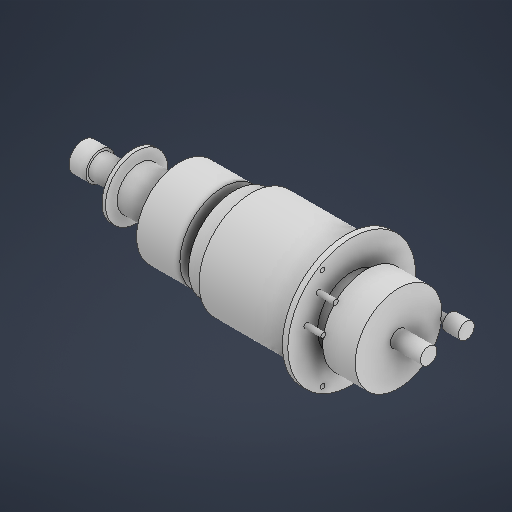
# Autodesk Inventor part: STI NGC Cryocooler
Saved by Autodesk Inventor 2026 (Build 300175050, 175E)
## iProperties
Created: 2024-04-30
Part Number: STI NGC Cryocooler
Material: Generic
Document SubType Name: Modeling
Designer: incep
Density: 1 g/cm^3
Appearance: Default
Author: incep
Autodesk Inventor part; units mm, degrees
ref_plane "YZ Plane" through (0, 0, 0) normal (1, 0, 0) x (0, 1, 0)
ref_plane "XZ Plane" through (0, 0, 0) normal (0, 1, 0) x (-1, 0, 0)
ref_plane "XY Plane" through (0, 0, 0) normal (0, 0, 1) x (1, 0, 0)
sketch "Sketch1" plane through (0, 0, 0) normal (0, 1, 0) x (-1, 0, 0)
  line L0 (0, 0) -> (-303.89, 0)
  line L1 (0, 0) -> (0, -10.5)
  line L2 (0, -10.5) -> (-94.6, -10.5)
  line L3 (-94.6, -10.5) -> (-94.6, -17.1)
  line L4 (-94.6, -17.1) -> (-46.4, -17.1)
  line L5 (-46.4, -17.1) -> (-46.4, -20.31)
  line L6 (-46.4, -20.31) -> (-43.9, -20.31)
  line L7 (-43.9, -20.31) -> (-43.9, -27.45)
  line L8 (-43.9, -27.45) -> (-47, -27.45)
  line L9 (-47, -27.45) -> (-48.9, -19.05)
  line L10 (-48.9, -19.05) -> (-84.8, -19.05)
  line L11 (-84.8, -19.05) -> (-84.8, -37.85)
  line L12 (-84.8, -37.85) -> (-122.9, -37.85)
  line L13 (-122.9, -37.85) -> (-122.9, -25.55)
  line L14 (-122.9, -25.55) -> (-132.9, -40.25)
  line L15 (-132.9, -40.25) -> (-132.9, -40.25)
  line L16 (-132.9, -40.25) -> (-147.9, -40.25)
  line L17 (-147.9, -40.25) -> (-147.9, -46)
  line L18 (-147.9, -46) -> (-150, -46)
  line L19 (-150, -46) -> (-150, -46)
  line L20 (-150, -46) -> (-231.4, -46)
  line L21 (-231.4, -46) -> (-231.4, -56.15)
  line L22 (-231.4, -56.15) -> (-236.2, -56.15)
  line L23 (-236.2, -56.15) -> (-236.2, 0)
  line L24 (-248.9, 0) -> (-248.9, -38.15)
  line L25 (-248.9, -38.15) -> (-277.4, -38.15)
  line L26 (-277.4, -38.15) -> (-277.4, -7.165)
  line L27 (-277.4, -7.165) -> (-303.89, -7.165)
  line L28 (-303.89, -7.165) -> (-303.89, 0)
  line L29 (0, -10.5) -> (0, -12.55)
  line L30 (0, -12.55) -> (-15, -12.55)
  line L31 (-15, -12.55) -> (-15, -10.5)
  line L32 (-236.2, 0) -> (-248.9, 0)
  line L33 (-248.9, 0) -> (-248.9, -30)
  line L34 (-248.9, -30) -> (-236.2, -30)
  line L35 (-236.2, -30) -> (-236.2, 0)
  dimension "d0" = 303.89
  dimension "d1" = 10.5
  dimension "d2" = 94.6
  dimension "d3" = 6.6
  dimension "d4" = 48.2
  dimension "d5" = 3.21
  dimension "d6" = 2.5
  dimension "d7" = 27.45
  dimension "d8" = 3.1
  dimension "d9" = 5
  dimension "d10" = 19.05
  dimension "d11" = 37.8
  dimension "d12" = 37.85
  dimension "d13" = 38.1
  dimension "d14" = 12.3
  dimension "d16" = 10
  dimension "d17" = 40.25
  dimension "d18" = 40.25
  dimension "d19" = 15
  dimension "d20" = 46
  dimension "d21" = 2.1
  dimension "d22" = 46
  dimension "d23" = 98.5
  dimension "d24" = 56.15
  dimension "d25" = 103.3
  dimension "d26" = 12.7
  dimension "d27" = 144.5
  dimension "d28" = 38.15
  dimension "d29" = 90
  dimension "d30" = 7.165
  dimension "d31" = 26.49
  dimension "d54" = 15
  dimension "d55" = 12.55
  dimension "d56" = 30
  constraints: 72 end point, 14 perpendicular, 9 vertical, 5 horizontal, 4 parallel, 4 point on line, 1 collinear
  measures "d0" distance of L0.start L0.end
  measures "d1" distance of L0.start L1.end
  measures "d2" distance of L1.end L2.end
  measures "d3" distance of L2.end L3.end
  measures "d4" distance of L3.end L4.end
  measures "d5" distance of L4.end L5.end
  measures "d6" distance of L5.end L6.end
  measures "d7" vertical distance of L0.start L7.end
  measures "d8" distance of L7.end L8.end
  measures "d9" distance from line of L9.end L7
  measures "d10" distance from line of L10 L0.start
  measures "d11" distance from line of L11 L8.end
  measures "d12" distance from line of L0.start L12
  measures "d13" distance of L11.end L12.end
  measures "d14" distance of L12.end L13.end
  measures "d16" distance between parallel lines of L15 L13
  measures "d17" distance from line of L14.end L0
  measures "d18" distance between parallel lines of L0 L16
  measures "d19" distance of L15.end L16.end
  measures "d20" distance between parallel lines of L0 L18
  measures "d21" distance of L17.end L18.end
  measures "d22" distance between parallel lines of L0 L20
  measures "d23" distance from line of L20.end L15
  measures "d24" distance between parallel lines of L0 L22
  measures "d25" distance between parallel lines of L23 L15
  measures "d26" distance between parallel lines of L24 L23
  measures "d27" distance from line of L25.end L15
  measures "d28" distance between parallel lines of L0 L25
  measures "d29" angle of L27 L26
  measures "d30" distance of L27.end L0.end
  measures "d31" distance of L26.end L27.end
  measures "d54" distance of L29.end L30.end
  measures "d55" distance between parallel lines of L0 L30
  measures "d56" distance between parallel lines of L34 L0
revolve "Revolution1" add sketch "Sketch1" angle 360 about axis through (0, 0, 0) along (1, 0, 0)
sketch "Sketch6" plane through (236.2, 0, 0) normal (1, 0, 0) x (0, 0, -1)
  line L0 (-25.5477, -44.25) -> (-25.5477, 44.25)
  line L1 (-25.5477, 44.25) -> (51.0955, 0)
  line L2 (51.0955, 0) -> (-25.5477, -44.25)
  circle A0 centre (51.0955, 0) radius 2
  circle A1 centre (-25.5477, -44.25) radius 2
  circle A2 centre (-25.5477, 44.25) radius 2
  point P0 (0, 0)
  point P1 (0, 0)
  dimension "d57" = 4
  dimension "d58" = 88.5
  constraints: 6 end point, 4 coincident, 3 centre point, 2 equal radius, 1 vertical, 7 other
  measures "d57" diameter of A0
  measures "d58" distance of L1.end L0.start
extrude "Extrusion3" cut sketch "Sketch6" against normal up to surface (4.8 mm away) contours L2 A1 L0 | L0 A1 L2 | A2 L1 L0 | L0 L1 A2 | A0 L1 L2 | L2 L1 A0
sketch "Sketch7" plane through (236.2, 0, 0) normal (1, 0, 0) x (0, 0, -1)
  circle A0 centre (0, 0) radius 30 projected
  circle A1 centre (0, 0) radius 41 construction
  circle A2 centre (-29.0395, 28.9432) radius 2.15
  circle A3 centre (-39.9405, 9.2603) radius 2.15
  circle A4 centre (-25.5477, 44.25) radius 2 projected
  dimension "d61" = 11
  dimension "d62" = 4.3
  dimension "d63" = 22.5
  dimension "d64" = 15.7
  constraints: 3 centre point, 2 point on circle, 1 equal radius
  measures "d61" radial gap between concentric circles of A1 A0
  measures "d62" diameter of A2
  measures "d63" distance of A3.centre A2.centre
  measures "d64" distance of A2.centre A4.centre
extrude "Extrusion4" add sketch "Sketch7" along normal blind 15 contours A2 | A3
sketch "Sketch8" plane through (236.2, 0, 0) normal (1, 0, 0) x (0, 0, -1)
  circle A0 centre (0, 0) radius 30 projected
  circle A1 centre (0, 0) radius 40 construction
  circle A2 centre (39.7956, -4.0388) radius 3.05
  circle A3 centre (51.0955, 0) radius 2 projected
  dimension "d67" = 10
  dimension "d68" = 6.1
  dimension "d69" = 12
  constraints: 1 centre point, 3 other
  measures "d68" diameter of A2
  measures "d69" distance of A2.centre A3.centre
extrude "Extrusion5" add sketch "Sketch8" along normal blind 61 contours A2
sketch "Sketch9" plane through (297.2, -4.0388, -39.7956) normal (1, 0, 0) x (0, 0, -1)
  circle A0 centre (0, 0) radius 3.05 projected
  circle A1 centre (0, 0) radius 7
  point P0 (-39.7956, 4.0388)
  dimension "d72" = 14
  constraints: 1 centre point, 1 coincident
  measures "d72" diameter of A1
extrude "Extrusion6" add sketch "Sketch9" against normal blind 14 contours A0 | A1
body "Solid1"
